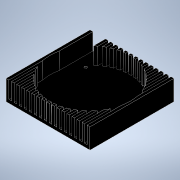
# Autodesk Inventor part: CPU_FPGA Cooler_for_delta_45mm
Saved by Autodesk Inventor 2021 (Build 250183000, 183)
## iProperties
Created: 2024-12-11
Part Number: CPU_FPGA Cooler_for_delta_45mm
Material: Aluminium 6061
Document SubType Name: Modeling
Designer: WS
Density: 2.7 g/cm^3
Appearance: Eloxiert - Schwarz
Author: WS
Autodesk Inventor part; units mm, degrees
ref_plane "YZ Plane" through (0, 0, 0) normal (1, 0, 0) x (0, 1, 0)
ref_plane "XZ Plane" through (0, 0, 0) normal (0, 1, 0) x (-1, 0, 0)
ref_plane "XY Plane" through (0, 0, 0) normal (0, 0, 1) x (1, 0, 0)
sketch "Skizze1" plane through (0, 0, 0) normal (0, 1, 0) x (-1, 0, 0)
  line L0 (0, 0) -> (50, 0)
  line L1 (50, 0) -> (50, -50)
  line L2 (50, -50) -> (0, -50)
  line L3 (0, -50) -> (0, 0)
  dimension "d0" = 50
  dimension "d1" = 50
  constraints: 8 end point, 2 parallel, 1 horizontal, 1 perpendicular
  measures "d0" distance of L1.end L2.end
  measures "d1" distance of L0.end L1.end
extrude "Extrusion1" add sketch "Skizze1" along normal blind 12
sketch "Skizze2" plane through (0, 12, 0) normal (0, 1, 0) x (1, 0, 0)
  circle A0 centre (-25, 25) radius 23.75
  line L0 (0, 0) -> (0, 50) projected
  line L1 (-50, 0) -> (0, 0) projected
  dimension "d4" = 47.5
  dimension "d5" = 25
  dimension "d6" = 25
  constraints: 1 centre point
  measures "d4" diameter of A0
  measures "d5" distance from line of L0 A0.centre
  measures "d6" distance from line of L1 A0.centre
extrude "Extrusion2" cut sketch "Skizze2" against normal blind 10
sketch "Skizze3" plane through (-50, 0, 0) normal (0, 0, 1) x (1, 0, 0)
  line L0 (0, 12) -> (50, 12) projected
  line L1 (1.75, 12) -> (3.25, 12)
  line L2 (3.25, 12) -> (3.25, 2)
  line L3 (3.25, 2) -> (1.75, 2)
  line L4 (1.75, 2) -> (1.75, 12)
  line L5 (0, 0) -> (0, 12) projected
  point P0 (50, 0)
  dimension "d9" = 1.5
  dimension "d10" = 10
  dimension "d11" = 1.75
  constraints: 8 end point, 2 parallel, 1 horizontal, 1 perpendicular, 1 point on line
  measures "d9" distance of L2.end L3.end
  measures "d10" distance of L1.end L2.end
  measures "d11" distance between parallel lines of L5 L4
extrude "Extrusion3" cut sketch "Skizze3" against normal through all
pattern_linear "Rechteckige Anordnung1" count 16 spacing 3 along (1, 0, 0) of "Extrusion3"
sketch "Skizze7" plane through (-25, 2, -25) normal (0, 1, 0) x (1, 0, 0)
  line L0 (0.4671, 0.3845) -> (-17.0187, 14.5442) construction
  line L1 (1.2537, 1.3559) -> (-16.2321, 15.5157)
  line L2 (-17.8054, 13.5728) -> (-0.3196, -0.5869)
  arc A0 (-0.3196, -0.5869) -> (1.2537, 1.3559) centre (0.4671, 0.3845) ccw
  arc A1 (-16.2321, 15.5157) -> (-17.8054, 13.5728) centre (-17.0187, 14.5442) ccw
  line L3 (0.4671, 0.3845) -> (22.9671, 0.3845) construction
  point P0 (25, -25)
  point P1 (-8.2758, 7.4644)
  dimension "d29" = 141
  dimension "d30" = 2.5
  dimension "d31" = 22.5
  constraints: 10 end point, 4 point on circle, 4 tangent, 2 centre point, 1 coincident, 1 equal length, 1 horizontal, 1 midpoint, 1 parallel
  measures "d29" angle of L3 L0
  measures "d30" diameter of A1
  measures "d31" distance of L0.start L0.end
hole "Bohrung1" at (-42.0187, 2, -39.5442) direction (0, -1, 0) diameter 1.6 end through all
pattern_circular "Runde Anordnung1" count 3 over 360 about axis through (-25, 12, -25) along (0, -1, 0) of "Bohrung1"
thread "Gewinde1" size "M2x0.4" class "6H" standard "ANSI Metric M Profile" full length
thread "Gewinde2" size "M2x0.4" class "6H" standard "ANSI Metric M Profile" full length
thread "Gewinde3" size "M2x0.4" class "6H" standard "ANSI Metric M Profile" full length
sketch "Skizze10" plane through (0, 12, 0) normal (0, 1, 0) x (1, 0, 0)
  arc A0 (-2.5, 17.3965) -> (-2.5, 32.6035) centre (-25, 25) ccw projected
  arc A1 (-2.5, 17.3965) -> (-1.75, 15.4606) centre (20, 25) ccw projected
  arc A2 (-1.75, 34.5394) -> (-2.5, 32.6035) centre (20, 25) ccw projected
  arc A3 (-1.75, 15.4606) -> (-2.5, 17.3965) centre (20, 25) ccw projected
  line L0 (-1.75, 34.5394) -> (-1.75, 15.4606)
  point P0 (0, 0)
  point P1 (-1.75, 20.1523)
  point P2 (-1.75, 29.8477)
  constraints: 2 end point, 1 vertical
extrude "Extrusion9" cut sketch "Skizze10" against normal up to surface (10 mm away) contours A0 L0 A1 | A2 L0 A0
sketch "Skizze11" plane through (0, 12, 0) normal (0, 1, 0) x (1, 0, 0)
  line L0 (-42.25, 41.3248) -> (-42.25, 50) projected
  line L1 (-42.25, 50) -> (-43.75, 50) projected
  line L2 (-43.75, 50) -> (-43.75, 39.5774) projected
  arc A0 (-42.25, 41.3248) -> (-43.75, 39.5774) centre (-25, 25) ccw projected
  line L3 (-39.25, 44) -> (-39.25, 50) projected
  line L4 (-39.25, 50) -> (-40.75, 50) projected
  line L5 (-40.75, 50) -> (-40.75, 42.7764) projected
  arc A1 (-39.25, 44) -> (-40.75, 42.7764) centre (-25, 25) ccw projected
  line L6 (-45.25, 37.4097) -> (-45.25, 50) projected
  line L7 (-45.25, 50) -> (-46.75, 50) projected
  line L8 (-46.75, 50) -> (-46.75, 34.5394) projected
  arc A2 (-45.25, 37.4097) -> (-46.75, 34.5394) centre (-25, 25) ccw projected
  point P0 (0, 0)
extrude "Extrusion11" cut sketch "Skizze11" against normal up to surface (10 mm away) contours A0 L2 L1 L0 | A2 L8 L7 L6
